Autodesk Inventor part; units mm, degrees
(part 2 of 2)
sketch "Sketch39" plane through (0, 25, 0) normal (0, 1, 0) x (1, 0, 0)
  line L0 (-75.5, 3.9) -> (-75.5, 131.7) projected
  line L1 (0, 3.9) -> (-85.5, 3.9) projected
  line L2 (-75.5, 131.7) -> (-71.5, 131.7)
  line L3 (-71.5, 131.7) -> (-71.5, 3.9)
  line L4 (-71.5, 3.9) -> (-75.5, 3.9)
  line L5 (-75.5, 3.9) -> (-75.5, 131.7)
  line L6 (-10, 3.9) -> (-10, 131.7) projected
  line L7 (-10, 131.7) -> (-14, 131.7)
  line L8 (-14, 131.7) -> (-14, 3.9)
  line L9 (-14, 3.9) -> (-10, 3.9)
  line L10 (-10, 3.9) -> (-10, 131.7)
  line L11 (-59.7793, 8.9543) -> (-63.625, 12.8) projected
  line L12 (-59.7793, 8.9543) -> (-57.7793, 8.9543)
  line L13 (-57.7793, 8.9543) -> (-57.7793, 6.9543)
  line L14 (-57.7793, 6.9543) -> (-59.7793, 6.9543)
  line L15 (-59.7793, 6.9543) -> (-59.7793, 8.9543)
  line L16 (-48.0957, 8.9543) -> (-44.25, 12.8) projected
  line L17 (-48.0957, 8.9543) -> (-50.0957, 8.9543)
  line L18 (-50.0957, 8.9543) -> (-50.0957, 3.9)
  line L19 (-50.0957, 3.9) -> (-48.0957, 3.9)
  line L20 (-48.0957, 3.9) -> (-48.0957, 8.9543)
  line L21 (0, 131.7) -> (-85.5, 131.7) projected
  line L22 (-50.0957, 3.9) -> (-57.7793, 3.9)
  line L23 (-57.7793, 3.9) -> (-57.7793, 131.7)
  line L24 (-57.7793, 131.7) -> (-50.0957, 131.7)
  line L25 (-50.0957, 131.7) -> (-50.0957, 3.9)
  line L26 (-38.4043, 8.9543) -> (-42.25, 12.8) projected
  line L27 (-38.4043, 8.9543) -> (-35.962, 8.9543)
  line L28 (-35.962, 8.9543) -> (-35.962, 3.9)
  line L29 (-35.962, 3.9) -> (-38.4043, 3.9)
  line L30 (-38.4043, 3.9) -> (-38.4043, 8.9543)
  line L31 (-26.7044, 8.9543) -> (-28.7044, 8.9543)
  line L32 (-28.7044, 8.9543) -> (-28.7044, 3.9)
  line L33 (-28.7044, 3.9) -> (-26.7044, 3.9)
  line L34 (-26.7044, 3.9) -> (-26.7044, 8.9543)
  line L35 (-35.962, 3.9) -> (-28.7044, 3.9)
  line L36 (-28.7044, 3.9) -> (-28.7044, 131.7)
  line L37 (-28.7044, 131.7) -> (-35.962, 131.7)
  line L38 (-35.962, 131.7) -> (-35.962, 3.9)
  line L39 (-69.4707, 126.6457) -> (-65.625, 122.8) projected
  line L40 (-69.4707, 126.6457) -> (-71.5, 126.6457)
  line L41 (-71.5, 126.6457) -> (-71.5, 128.6457)
  line L42 (-71.5, 128.6457) -> (-69.4707, 128.6457)
  line L43 (-69.4707, 128.6457) -> (-69.4707, 126.6457)
  line L44 (-85.5, 131.7) -> (-75.5, 131.7) projected
  line L45 (-75.5, 131.7) -> (-10, 131.7)
  line L46 (-10, 131.7) -> (-10, 128.6457)
  line L47 (-10, 128.6457) -> (-75.5, 128.6457)
  line L48 (-75.5, 128.6457) -> (-75.5, 131.7)
  line L49 (-75.5, 3.9) -> (-14, 3.9)
  line L50 (-14, 3.9) -> (-14, 6.9543)
  line L51 (-14, 6.9543) -> (-75.5, 6.9543)
  line L52 (-75.5, 6.9543) -> (-75.5, 3.9)
  point P0 (0, 0)
  point P1 (-28.7044, 128.6457)
  point P2 (-14, 128.6457)
  point P3 (-28.7044, 6.9543)
  point P4 (-50.0957, 128.6457)
  point P5 (-35.962, 128.6457)
  point P6 (-35.962, 6.9543)
  point P7 (-50.0957, 6.9543)
  point P8 (-57.7793, 128.6457)
  point P9 (-71.5, 6.9543)
  dimension "d181" = 4
  dimension "d182" = 4
  dimension "d183" = 2
  dimension "d184" = 2
  dimension "d185" = 2
  dimension "d186" = 2
  dimension "d187" = 2
  constraints: 88 end point, 22 parallel, 14 point on line, 11 horizontal, 11 perpendicular
  measures "d181" distance of L3.end L4.end
  measures "d182" distance of L9.end L8.end
  measures "d183" distance of L13.end L14.end
  measures "d184" distance of L12.end L13.end
  measures "d185" distance of L19.end L18.end
  measures "d186" distance of L33.end L32.end
  measures "d187" distance of L40.end L41.end
extrude "Extrusion36" cut sketch "Sketch39" against normal blind 20 contours L0 L51 L3 L1 | L0 L47 L3 L51 | L3 L51 L14 L23 L1 | L0 L2 L3 L47 | L23 L51 L18 L1 | L3 L21 L23 L47 L42 | L18 L51 L20 L1 | L13 L23 L47 L25 L18 L51 | L20 L51 L30 L1 | L21 L25 L47 L23 | L30 L51 L28 L1 | L21 L38 L47 L25 | L28 L51 L32 L1 | L21 L36 L47 L38 | L47 L36 L32 L51 L28 L38 | L32 L51 L34 L1 | L21 L8 L47 L36 | L34 L51 L8 L1 | L7 L6 L47 L8 | L47 L6 L1 L8
sketch "Sketch41" plane through (0, 25, 0) normal (0, 1, 0) x (1, 0, 0)
  line L0 (-77.7032, 134.0912) -> (-53.8399, 134.0912)
  line L1 (-53.8399, 134.0912) -> (-53.8399, -1.2645)
  line L2 (-53.8399, -1.2645) -> (-77.7032, -1.2645)
  line L3 (-77.7032, -1.2645) -> (-77.7032, 134.0912)
  line L4 (-30.9546, 135.8516) -> (-10.2209, 135.8516)
  line L5 (-10.2209, 135.8516) -> (-10.2209, -6.5457)
  line L6 (-10.2209, -6.5457) -> (-30.9546, -6.5457)
  line L7 (-30.9546, -6.5457) -> (-30.9546, 135.8516)
  point P0 (0, 0)
  constraints: 16 end point, 4 parallel, 2 horizontal, 2 perpendicular
extrude "Extrusion37" cut sketch "Sketch41" against normal blind 20
sketch "Sketch42" plane through (0, 5, 0) normal (0, 1, 0) x (1, 0, 0)
  line L0 (-72.732, 126.4568) -> (-55.877, 126.4568)
  line L1 (-55.877, 126.4568) -> (-55.877, 7.7978)
  line L2 (-55.877, 7.7978) -> (-72.732, 7.7978)
  line L3 (-72.732, 7.7978) -> (-72.732, 126.4568)
  line L4 (-10.2563, 126.4568) -> (-31.3812, 126.4568)
  line L5 (-31.3812, 126.4568) -> (-31.3812, 7.7978)
  line L6 (-31.3812, 7.7978) -> (-10.2563, 7.7978)
  line L7 (-10.2563, 7.7978) -> (-10.2563, 126.4568)
  point P0 (0, 0)
  constraints: 16 end point, 4 parallel, 2 horizontal, 2 perpendicular, 2 point on line
extrude "Extrusion38" add sketch "Sketch42" against normal blind 5
sketch "Sketch43" plane through (0, 5, 0) normal (0, 1, 0) x (1, 0, 0)
  line L0 (0, 131.7) -> (-85.5, 131.7) projected
  line L1 (-85.5, 131.7) -> (-82.446, 131.7)
  line L2 (-82.446, 131.7) -> (-82.446, 128.646)
  line L3 (-82.446, 128.646) -> (-85.5, 128.646)
  line L4 (-85.5, 128.646) -> (-85.5, 131.7)
  line L5 (0, 131.7) -> (-3.054, 131.7)
  line L6 (-3.054, 131.7) -> (-3.054, 128.646)
  line L7 (-3.054, 128.646) -> (0, 128.646)
  line L8 (0, 128.646) -> (0, 131.7)
  line L9 (0, 3.9) -> (-3.054, 3.9)
  line L10 (-3.054, 3.9) -> (-3.054, 6.954)
  line L11 (-3.054, 6.954) -> (0, 6.954)
  line L12 (0, 6.954) -> (0, 3.9)
  line L13 (-85.5, 3.9) -> (-82.446, 3.9)
  line L14 (-82.446, 3.9) -> (-82.446, 6.954)
  line L15 (-82.446, 6.954) -> (-85.5, 6.954)
  line L16 (-85.5, 6.954) -> (-85.5, 3.9)
  line L17 (-82.446, 6.954) -> (-3.054, 6.954)
  line L18 (-3.054, 6.954) -> (-3.054, 128.646)
  line L19 (-3.054, 128.646) -> (-82.446, 128.646)
  line L20 (-82.446, 128.646) -> (-82.446, 6.954)
  line L21 (-82.446, 128.646) -> (-68.312, 128.646)
  line L22 (-68.312, 128.646) -> (-68.312, 6.954)
  line L23 (-68.312, 6.954) -> (-82.446, 6.954)
  line L24 (-82.446, 6.954) -> (-82.446, 128.646)
  line L25 (-3.054, 128.646) -> (-17.188, 128.646)
  line L26 (-17.188, 128.646) -> (-17.188, 6.954)
  line L27 (-17.188, 6.954) -> (-3.054, 6.954)
  line L28 (-3.054, 6.954) -> (-3.054, 128.646)
  point P0 (0, 0)
  dimension "d194" = 3.054
  dimension "d195" = 3.054
  dimension "d196" = 3.054
  dimension "d197" = 3.054
  dimension "d198" = 3.054
  dimension "d199" = 3.054
  dimension "d200" = 3.054
  dimension "d201" = 3.054
  dimension "d202" = 14.134
  dimension "d203" = 14.134
  constraints: 56 end point, 14 parallel, 7 horizontal, 7 perpendicular, 2 point on line
  measures "d194" distance of L2.end L3.end
  measures "d195" distance of L1.end L2.end
  measures "d196" distance of L7.end L6.end
  measures "d197" distance of L6.end L5.end
  measures "d198" distance of L10.end L11.end
  measures "d199" distance of L9.end L10.end
  measures "d200" distance of L15.end L14.end
  measures "d201" distance of L14.end L13.end
  measures "d202" distance of L22.end L23.end
  measures "d203" distance of L27.end L26.end
extrude "Extrusion39" add sketch "Sketch43" along normal blind 20 contours L18 L17 L26 L19 | L19 L22 L17 L20
sketch "Sketch44" plane through (0, 25, 0) normal (0, 1, 0) x (1, 0, 0)
  point P0 (0, 0)
sketch "Sketch45" plane through (0, 25, 0) normal (0, 1, 0) x (1, 0, 0)
  line L0 (-42.25, 22.8) -> (-44.25, 22.8) projected
  line L1 (-2.93, 12.8) -> (-44.25, 12.8)
  line L2 (-44.25, 12.8) -> (-44.25, 22.8)
  line L3 (-44.25, 22.8) -> (-2.93, 22.8)
  line L4 (-2.93, 22.8) -> (-2.93, 12.8)
  line L5 (-42.25, 12.8) -> (-82.5029, 12.8)
  line L6 (-82.5029, 12.8) -> (-82.5029, 22.8)
  line L7 (-82.5029, 22.8) -> (-42.25, 22.8)
  line L8 (-42.25, 22.8) -> (-42.25, 12.8)
  line L9 (-42.25, 32.8) -> (-42.25, 42.8) projected
  line L10 (-42.25, 32.8) -> (-82.5029, 32.8)
  line L11 (-82.5029, 32.8) -> (-82.5029, 42.8)
  line L12 (-82.5029, 42.8) -> (-42.25, 42.8)
  line L13 (-42.25, 42.8) -> (-42.25, 32.8)
  line L14 (-44.25, 42.8) -> (-44.25, 32.8) projected
  line L15 (-3.054, 6.954) -> (-3.054, 128.646) projected
  line L16 (-44.25, 32.8) -> (-3.054, 32.8)
  line L17 (-3.054, 32.8) -> (-3.054, 42.8)
  line L18 (-3.054, 42.8) -> (-44.25, 42.8)
  line L19 (-44.25, 42.8) -> (-44.25, 32.8)
  line L20 (-44.25, 62.8) -> (-44.25, 52.8) projected
  line L21 (-44.25, 52.8) -> (-3.054, 52.8)
  line L22 (-3.054, 52.8) -> (-3.054, 62.8)
  line L23 (-3.054, 62.8) -> (-44.25, 62.8)
  line L24 (-44.25, 62.8) -> (-44.25, 52.8)
  line L25 (-44.25, 52.8) -> (-42.25, 52.8) projected
  line L26 (-42.25, 52.8) -> (-82.5029, 52.8)
  line L27 (-82.5029, 52.8) -> (-82.5029, 62.8)
  line L28 (-82.5029, 62.8) -> (-42.25, 62.8)
  line L29 (-42.25, 62.8) -> (-42.25, 52.8)
  line L30 (-44.25, 72.8) -> (-42.25, 72.8) projected
  line L31 (-44.25, 72.8) -> (-3.054, 72.8)
  line L32 (-3.054, 72.8) -> (-3.054, 82.8104)
  line L33 (-3.054, 82.8104) -> (-44.25, 82.8104)
  line L34 (-44.25, 82.8104) -> (-44.25, 72.8)
  line L35 (-42.25, 72.8) -> (-42.25, 82.8) projected
  line L36 (-42.25, 72.8) -> (-82.5029, 72.8)
  line L37 (-82.5029, 72.8) -> (-82.5029, 82.8104)
  line L38 (-82.5029, 82.8104) -> (-42.25, 82.8104)
  line L39 (-42.25, 82.8104) -> (-42.25, 72.8)
  line L40 (-44.25, 102.8) -> (-44.25, 92.8) projected
  line L41 (-44.25, 92.8) -> (-3.054, 92.8)
  line L42 (-3.054, 92.8) -> (-3.054, 102.8)
  line L43 (-3.054, 102.8) -> (-44.25, 102.8)
  line L44 (-44.25, 102.8) -> (-44.25, 92.8)
  line L45 (-42.25, 92.8) -> (-42.25, 102.8) projected
  line L46 (-82.446, 6.954) -> (-82.446, 128.646) projected
  line L47 (-42.25, 92.8) -> (-82.446, 92.8)
  line L48 (-82.446, 92.8) -> (-82.446, 102.8)
  line L49 (-82.446, 102.8) -> (-42.25, 102.8)
  line L50 (-42.25, 102.8) -> (-42.25, 92.8)
  line L51 (-42.25, 112.8) -> (-82.446, 112.8)
  line L52 (-82.446, 112.8) -> (-82.446, 122.8)
  line L53 (-82.446, 122.8) -> (-42.25, 122.8)
  line L54 (-42.25, 122.8) -> (-42.25, 112.8)
  line L55 (-44.25, 112.8) -> (-3.054, 112.8)
  line L56 (-3.054, 112.8) -> (-3.054, 122.8)
  line L57 (-3.054, 122.8) -> (-44.25, 122.8)
  line L58 (-44.25, 122.8) -> (-44.25, 112.8)
  line L59 (-17.188, 128.646) -> (-17.188, 6.954) projected
  line L60 (-3.054, 128.646) -> (-17.188, 128.646) projected
  line L61 (-17.188, 6.954) -> (-11.324, 6.954)
  line L62 (-11.324, 6.954) -> (-11.324, 128.646)
  line L63 (-11.324, 128.646) -> (-17.188, 128.646)
  line L64 (-17.188, 128.646) -> (-17.188, 6.954)
  line L65 (-82.446, 6.954) -> (-68.312, 6.954) projected
  line L66 (-68.312, 128.646) -> (-82.446, 128.646) projected
  line L67 (-68.312, 6.954) -> (-74.176, 6.954)
  line L68 (-74.176, 6.954) -> (-74.176, 128.646)
  line L69 (-74.176, 128.646) -> (-68.312, 128.646)
  line L70 (-68.312, 128.646) -> (-68.312, 6.954)
  line L71 (-82.446, 128.646) -> (-76.582, 128.646)
  line L72 (-76.582, 128.646) -> (-76.582, 6.954)
  line L73 (-76.582, 6.954) -> (-82.446, 6.954)
  line L74 (-82.446, 6.954) -> (-82.446, 128.646)
  line L75 (-17.188, 6.954) -> (-3.054, 6.954) projected
  line L76 (-3.054, 6.954) -> (-8.918, 6.954)
  line L77 (-8.918, 6.954) -> (-8.918, 128.646)
  line L78 (-8.918, 128.646) -> (-3.054, 128.646)
  line L79 (-3.054, 128.646) -> (-3.054, 6.954)
  point P0 (0, 0)
  point P1 (-76.582, 22.8)
  point P2 (-76.582, 12.8)
  point P3 (-74.176, 12.8)
  point P4 (-74.176, 22.8)
  point P5 (-76.582, 42.8)
  point P6 (-76.582, 32.8)
  point P7 (-74.176, 32.8)
  point P8 (-74.176, 42.8)
  point P9 (-76.582, 62.8)
  point P10 (-76.582, 52.8)
  point P11 (-74.176, 52.8)
  point P12 (-74.176, 62.8)
  point P13 (-76.582, 82.8104)
  point P14 (-76.582, 72.8)
  point P15 (-74.176, 72.8)
  point P16 (-74.176, 82.8104)
  point P17 (-76.582, 102.8)
  point P18 (-76.582, 92.8)
  point P19 (-74.176, 92.8)
  point P20 (-74.176, 102.8)
  point P21 (-76.582, 122.8)
  point P22 (-76.582, 112.8)
  point P23 (-74.176, 112.8)
  point P24 (-74.176, 122.8)
  point P25 (-8.918, 112.8)
  point P26 (-8.918, 122.8)
  point P27 (-11.324, 122.8)
  point P28 (-11.324, 112.8)
  point P29 (-8.918, 92.8)
  point P30 (-8.918, 102.8)
  point P31 (-11.324, 102.8)
  point P32 (-11.324, 92.8)
  point P33 (-8.918, 72.8)
  point P34 (-8.918, 82.8104)
  point P35 (-11.324, 82.8104)
  point P36 (-11.324, 72.8)
  point P37 (-8.918, 52.8)
  point P38 (-8.918, 62.8)
  point P39 (-11.324, 62.8)
  point P40 (-11.324, 52.8)
  point P41 (-8.918, 32.8)
  point P42 (-8.918, 42.8)
  point P43 (-11.324, 42.8)
  point P44 (-11.324, 32.8)
  point P45 (-8.918, 12.8)
  point P46 (-8.918, 22.8)
  point P47 (-11.324, 22.8)
  point P48 (-11.324, 12.8)
  dimension "d206" = 5.864
  dimension "d207" = 5.864
  dimension "d208" = 5.864
  dimension "d209" = 5.864
  constraints: 128 end point, 32 parallel, 21 point on line, 16 horizontal, 16 perpendicular
  measures "d206" distance of L63.end L62.end
  measures "d207" distance of L68.end L69.end
  measures "d208" distance of L72.end L73.end
  measures "d209" distance of L77.end L78.end
extrude "Extrusion40" cut sketch "Sketch45" against normal blind 100 contours L3 L77 L1 L62 | L68 L5 L72 L7 | L62 L18 L77 L16 | L10 L72 L12 L68 | L62 L23 L77 L21 | L26 L72 L28 L68 | L62 L33 L77 L31 | L36 L72 L38 L68 | L62 L43 L77 L41 | L47 L72 L49 L68 | L62 L57 L77 L55 | L51 L72 L53 L68
chamfer "Chamfer6" distance 5 distance2 15 1 edges at (-8.918, 25, -17.8) measured on face at (-8.418, 25, -17.8)
chamfer "Chamfer7" distance 5 distance2 15 1 edges at (-8.918, 25, -37.8) measured on face at (-8.418, 25, -37.8)
chamfer "Chamfer8" distance 5 distance2 15 1 edges at (-8.918, 25, -57.8) measured on face at (-8.418, 25, -57.8)
chamfer "Chamfer9" distance 5 distance2 15 1 edges at (-8.918, 25, -77.8052) measured on face at (-8.418, 25, -77.8052)
chamfer "Chamfer10" distance 5 distance2 15 1 edges at (-8.918, 25, -97.8) measured on face at (-8.418, 25, -97.8)
chamfer "Chamfer11" distance 5 distance2 15 1 edges at (-8.918, 25, -117.8) measured on face at (-8.418, 25, -117.8)
chamfer "Chamfer12" distance 5 distance2 15 1 edges at (-11.324, 25, -117.8) measured on face at (-11.824, 25, -117.8)
chamfer "Chamfer13" distance 5 distance2 15 1 edges at (-11.324, 25, -97.8) measured on face at (-11.824, 25, -97.8)
chamfer "Chamfer14" distance 5 distance2 15 1 edges at (-11.324, 25, -77.8052) measured on face at (-11.824, 25, -77.8052)
chamfer "Chamfer15" distance 5 distance2 15 1 edges at (-11.324, 25, -57.8) measured on face at (-11.824, 25, -57.8)
chamfer "Chamfer16" distance 5 distance2 15 1 edges at (-11.324, 25, -37.8) measured on face at (-11.824, 25, -37.8)
chamfer "Chamfer17" distance 5 distance2 15 1 edges at (-11.324, 25, -17.8) measured on face at (-11.824, 25, -17.8)
chamfer "Chamfer18" distance 5 distance2 15 1 edges at (-74.176, 25, -17.8) measured on face at (-73.676, 25, -17.8)
chamfer "Chamfer19" distance 5 distance2 15 1 edges at (-76.582, 25, -17.8) measured on face at (-77.082, 25, -17.8)
chamfer "Chamfer20" distance 5 distance2 15 1 edges at (-74.176, 25, -37.8) measured on face at (-73.676, 25, -37.8)
chamfer "Chamfer21" distance 5 distance2 15 1 edges at (-76.582, 25, -37.8) measured on face at (-77.082, 25, -37.8)
chamfer "Chamfer22" distance 5 distance2 15 1 edges at (-76.582, 25, -57.8) measured on face at (-77.082, 25, -57.8)
chamfer "Chamfer23" distance 5 distance2 15 1 edges at (-74.176, 25, -57.8) measured on face at (-73.676, 25, -57.8)
chamfer "Chamfer24" distance 5 distance2 15 1 edges at (-74.176, 25, -77.8052) measured on face at (-73.676, 25, -77.8052)
chamfer "Chamfer25" distance 5 distance2 15 1 edges at (-76.582, 25, -77.8052) measured on face at (-77.082, 25, -77.8052)
chamfer "Chamfer26" distance 5 distance2 15 1 edges at (-74.176, 25, -97.8) measured on face at (-73.676, 25, -97.8)
chamfer "Chamfer27" distance 5 distance2 15 1 edges at (-76.582, 25, -97.8) measured on face at (-77.082, 25, -97.8)
chamfer "Chamfer28" distance 5 distance2 15 1 edges at (-74.176, 25, -117.8) measured on face at (-73.676, 25, -117.8)
chamfer "Chamfer29" distance 5 distance2 15 1 edges at (-76.582, 25, -117.8) measured on face at (-77.082, 25, -117.8)
chamfer "Chamfer30" distance 1 distance2 15 3 edges at (-13.824, 25, -12.8) (-10.121, 25, -12.8) (-6.418, 25, -12.8) measured on face at (-13.824, 25, -12.3) measured on face at (-10.121, 25, -12.3) measured on face at (-6.418, 25, -12.3)
chamfer "Chamfer31" distance 1 distance2 15 3 edges at (-6.418, 25, -22.8) (-10.121, 25, -22.8) (-13.824, 25, -22.8) measured on face at (-13.824, 25, -23.3) measured on face at (-10.121, 25, -23.3) measured on face at (-6.418, 25, -23.3)
chamfer "Chamfer32" distance 1 distance2 15 3 edges at (-13.824, 25, -32.8) (-10.121, 25, -32.8) (-6.418, 25, -32.8) measured on face at (-10.121, 25, -32.3) measured on face at (-6.418, 25, -32.3) measured on face at (-13.824, 25, -32.3)
chamfer "Chamfer33" distance 1 distance2 15 3 edges at (-6.418, 25, -42.8) (-10.121, 25, -42.8) (-13.824, 25, -42.8) measured on face at (-10.121, 25, -43.3) measured on face at (-6.418, 25, -43.3) measured on face at (-13.824, 25, -43.3)
chamfer "Chamfer34" distance 1 distance2 15 3 edges at (-13.824, 25, -62.8) (-10.121, 25, -62.8) (-6.418, 25, -62.8) measured on face at (-6.418, 25, -63.3) measured on face at (-13.824, 25, -63.3) measured on face at (-10.121, 25, -63.3)
chamfer "Chamfer35" distance 1 distance2 15 3 edges at (-6.418, 25, -52.8) (-10.121, 25, -52.8) (-13.824, 25, -52.8) measured on face at (-6.418, 25, -52.3) measured on face at (-13.824, 25, -52.3) measured on face at (-10.121, 25, -52.3)
chamfer "Chamfer36" distance 1 distance2 15 3 edges at (-13.824, 25, -72.8) (-10.121, 25, -72.8) (-6.418, 25, -72.8) measured on face at (-6.418, 25, -72.3) measured on face at (-13.824, 25, -72.3) measured on face at (-10.121, 25, -72.3)
chamfer "Chamfer37" distance 1 distance2 15 3 edges at (-6.418, 25, -82.8104) (-10.121, 25, -82.8104) (-13.824, 25, -82.8104) measured on face at (-13.824, 25, -83.3104) measured on face at (-10.121, 25, -83.3104) measured on face at (-6.418, 25, -83.3104)
chamfer "Chamfer38" distance 1 distance2 15 3 edges at (-13.824, 25, -92.8) (-10.121, 25, -92.8) (-6.418, 25, -92.8) measured on face at (-13.824, 25, -92.3) measured on face at (-10.121, 25, -92.3) measured on face at (-6.418, 25, -92.3)
chamfer "Chamfer39" distance 1 distance2 15 3 edges at (-6.418, 25, -102.8) (-10.121, 25, -102.8) (-13.824, 25, -102.8) measured on face at (-13.824, 25, -103.3) measured on face at (-10.121, 25, -103.3) measured on face at (-6.418, 25, -103.3)
chamfer "Chamfer40" distance 1 distance2 15 3 edges at (-13.824, 25, -112.8) (-10.121, 25, -112.8) (-6.418, 25, -112.8) measured on face at (-6.418, 25, -112.3) measured on face at (-13.824, 25, -112.3) measured on face at (-10.121, 25, -112.3)
chamfer "Chamfer41" distance 1 distance2 15 3 edges at (-6.418, 25, -122.8) (-10.121, 25, -122.8) (-13.824, 25, -122.8) measured on face at (-6.418, 25, -123.3) measured on face at (-13.824, 25, -123.3) measured on face at (-10.121, 25, -123.3)
chamfer "Chamfer42" distance 1 distance2 15 3 edges at (-79.082, 25, -12.8) (-75.379, 25, -12.8) (-71.676, 25, -12.8) measured on face at (-75.379, 25, -12.3) measured on face at (-71.676, 25, -12.3) measured on face at (-79.082, 25, -12.3)
chamfer "Chamfer43" distance 1 distance2 15 3 edges at (-71.676, 25, -22.8) (-75.379, 25, -22.8) (-79.082, 25, -22.8) measured on face at (-75.379, 25, -23.3) measured on face at (-71.676, 25, -23.3) measured on face at (-79.082, 25, -23.3)
chamfer "Chamfer44" distance 1 distance2 15 3 edges at (-79.082, 25, -42.8) (-75.379, 25, -42.8) (-71.676, 25, -42.8) measured on face at (-71.676, 25, -43.3) measured on face at (-75.379, 25, -43.3) measured on face at (-79.082, 25, -43.3)
chamfer "Chamfer45" distance 1 distance2 15 3 edges at (-71.676, 25, -32.8) (-75.379, 25, -32.8) (-79.082, 25, -32.8) measured on face at (-75.379, 25, -32.3) measured on face at (-71.676, 25, -32.3) measured on face at (-79.082, 25, -32.3)
chamfer "Chamfer46" distance 1 distance2 15 3 edges at (-71.676, 25, -52.8) (-75.379, 25, -52.8) (-79.082, 25, -52.8) measured on face at (-71.676, 25, -52.3) measured on face at (-75.379, 25, -52.3) measured on face at (-79.082, 25, -52.3)
chamfer "Chamfer47" distance 1 distance2 15 3 edges at (-79.082, 25, -62.8) (-75.379, 25, -62.8) (-71.676, 25, -62.8) measured on face at (-71.676, 25, -63.3) measured on face at (-75.379, 25, -63.3) measured on face at (-79.082, 25, -63.3)
chamfer "Chamfer48" distance 1 distance2 15 3 edges at (-79.082, 25, -72.8) (-75.379, 25, -72.8) (-71.676, 25, -72.8) measured on face at (-71.676, 25, -72.3) measured on face at (-75.379, 25, -72.3) measured on face at (-79.082, 25, -72.3)
chamfer "Chamfer49" distance 1 distance2 15 3 edges at (-71.676, 25, -82.8104) (-75.379, 25, -82.8104) (-79.082, 25, -82.8104) measured on face at (-71.676, 25, -83.3104) measured on face at (-79.082, 25, -83.3104) measured on face at (-75.379, 25, -83.3104)
chamfer "Chamfer50" distance 1 distance2 15 3 edges at (-79.082, 25, -92.8) (-75.379, 25, -92.8) (-71.676, 25, -92.8) measured on face at (-71.676, 25, -92.3) measured on face at (-75.379, 25, -92.3) measured on face at (-79.082, 25, -92.3)
chamfer "Chamfer51" distance 1 distance2 15 3 edges at (-71.676, 25, -102.8) (-75.379, 25, -102.8) (-79.082, 25, -102.8) measured on face at (-75.379, 25, -103.3) measured on face at (-71.676, 25, -103.3) measured on face at (-79.082, 25, -103.3)
chamfer "Chamfer52" distance 1 distance2 15 3 edges at (-79.082, 25, -112.8) (-75.379, 25, -112.8) (-71.676, 25, -112.8) measured on face at (-75.379, 25, -112.3) measured on face at (-79.082, 25, -112.3) measured on face at (-71.676, 25, -112.3)
chamfer "Chamfer53" distance 1 distance2 15 3 edges at (-71.676, 25, -122.8) (-75.379, 25, -122.8) (-79.082, 25, -122.8) measured on face at (-75.379, 25, -123.3) measured on face at (-79.082, 25, -123.3) measured on face at (-71.676, 25, -123.3)
sketch "Sketch46" plane through (0, 25, 0) normal (0, 1, 0) x (1, 0, 0)
  line L0 (-42.25, 12.8) -> (-42.25, 22.8) projected
  line L1 (-42.25, 22.8) -> (-44.25, 22.8) projected
  line L2 (-42.25, 12.8) -> (-44.25, 12.8)
  line L3 (-44.25, 12.8) -> (-44.25, 22.8)
  line L4 (-44.25, 22.8) -> (-42.25, 22.8)
  line L5 (-42.25, 22.8) -> (-42.25, 12.8)
  line L6 (-44.25, 32.8) -> (-42.25, 32.8) projected
  line L7 (-42.25, 42.8) -> (-44.25, 42.8) projected
  line L8 (-42.25, 32.8) -> (-44.25, 32.8)
  line L9 (-44.25, 32.8) -> (-44.25, 42.8)
  line L10 (-44.25, 42.8) -> (-42.25, 42.8)
  line L11 (-42.25, 42.8) -> (-42.25, 32.8)
  line L12 (-42.25, 52.8) -> (-42.25, 62.8) projected
  line L13 (-42.25, 52.8) -> (-44.25, 52.8)
  line L14 (-44.25, 52.8) -> (-44.25, 62.8)
  line L15 (-44.25, 62.8) -> (-42.25, 62.8)
  line L16 (-42.25, 62.8) -> (-42.25, 52.8)
  line L17 (-42.25, 72.8) -> (-42.25, 82.8) projected
  line L18 (-42.25, 72.8) -> (-44.25, 72.8)
  line L19 (-44.25, 72.8) -> (-44.25, 82.8)
  line L20 (-44.25, 82.8) -> (-42.25, 82.8)
  line L21 (-42.25, 82.8) -> (-42.25, 72.8)
  line L22 (-42.25, 92.8098) -> (-44.25, 92.8098)
  line L23 (-44.25, 92.8098) -> (-44.25, 102.7913)
  line L24 (-44.25, 102.7913) -> (-42.25, 102.7913)
  line L25 (-42.25, 102.7913) -> (-42.25, 92.8098)
  line L26 (-42.25, 112.8) -> (-42.25, 122.8) projected
  line L27 (-42.25, 112.8) -> (-44.25, 112.8)
  line L28 (-44.25, 112.8) -> (-44.25, 122.8)
  line L29 (-44.25, 122.8) -> (-42.25, 122.8)
  line L30 (-42.25, 122.8) -> (-42.25, 112.8)
  point P0 (0, 0)
  constraints: 48 end point, 12 parallel, 6 horizontal, 6 perpendicular, 5 point on line
sketch "Sketch47" plane through (0, 25, 0) normal (0, 1, 0) x (1, 0, 0)
  line L0 (-35.962, 6.9543) -> (-35.962, 128.6457) projected
  line L1 (-50.0957, 128.6457) -> (-50.0957, 6.9543) projected
  line L2 (-35.962, 6.9543) -> (-50.0957, 6.9543)
  line L3 (-50.0957, 6.9543) -> (-50.0957, 128.6457)
  line L4 (-50.0957, 128.6457) -> (-35.962, 128.6457)
  line L5 (-35.962, 128.6457) -> (-35.962, 6.9543)
  point P0 (0, 0)
  constraints: 8 end point, 2 parallel, 1 horizontal, 1 perpendicular
extrude "Extrusion41" add sketch "Sketch47" against normal blind 25
extrude "Extrusion42" cut sketch "Sketch46" against normal blind 25
chamfer "Chamfer54" distance 5 distance2 15 1 edges at (-44.25, 25, -17.8) measured on face at (-44.75, 25, -17.8)
chamfer "Chamfer55" distance 5 distance2 15 1 edges at (-42.25, 25, -17.8) measured on face at (-41.75, 25, -17.8)
chamfer "Chamfer56" distance 5 distance2 15 1 edges at (-42.25, 25, -37.8) measured on face at (-41.75, 25, -37.8)
chamfer "Chamfer57" distance 5 distance2 15 1 edges at (-44.25, 25, -37.8) measured on face at (-44.75, 25, -37.8)
chamfer "Chamfer58" distance 5 distance2 15 1 edges at (-42.25, 25, -57.8) measured on face at (-41.75, 25, -57.8)
chamfer "Chamfer59" distance 5 distance2 15 1 edges at (-44.25, 25, -57.8) measured on face at (-44.75, 25, -57.8)
chamfer "Chamfer60" distance 5 distance2 15 1 edges at (-42.25, 25, -77.8) measured on face at (-41.75, 25, -77.8)
chamfer "Chamfer61" distance 5 distance2 15 1 edges at (-44.25, 25, -77.8) measured on face at (-44.75, 25, -77.8)
chamfer "Chamfer62" distance 5 distance2 15 1 edges at (-42.25, 25, -97.8005)
chamfer "Chamfer63" distance 5 distance2 15 1 edges at (-44.25, 25, -97.8005)
chamfer "Chamfer64" distance 5 distance2 15 1 edges at (-42.25, 25, -117.8) measured on face at (-41.75, 25, -117.8)
chamfer "Chamfer65" distance 5 distance2 15 1 edges at (-44.25, 25, -117.8) measured on face at (-44.75, 25, -117.8)
chamfer "Chamfer66" distance 1 distance2 15 3 edges at (-39.75, 25, -12.8) (-43.25, 25, -12.8) (-46.75, 25, -12.8) measured on face at (-43.25, 25, -12.3) measured on face at (-46.75, 25, -12.3) measured on face at (-39.75, 25, -12.3)
chamfer "Chamfer67" distance 1 distance2 15 3 edges at (-46.75, 25, -22.8) (-43.25, 25, -22.8) (-39.75, 25, -22.8) measured on face at (-39.75, 25, -23.3) measured on face at (-46.75, 25, -23.3) measured on face at (-43.25, 25, -23.3)
chamfer "Chamfer68" distance 1 distance2 15 3 edges at (-46.75, 25, -32.8) (-43.25, 25, -32.8) (-39.75, 25, -32.8) measured on face at (-46.75, 25, -32.3) measured on face at (-43.25, 25, -32.3) measured on face at (-39.75, 25, -32.3)
chamfer "Chamfer69" distance 1 distance2 15 3 edges at (-39.75, 25, -42.8) (-43.25, 25, -42.8) (-46.75, 25, -42.8) measured on face at (-46.75, 25, -43.3) measured on face at (-43.25, 25, -43.3) measured on face at (-39.75, 25, -43.3)
chamfer "Chamfer70" distance 1 distance2 15 3 edges at (-46.75, 25, -52.8) (-43.25, 25, -52.8) (-39.75, 25, -52.8) measured on face at (-43.25, 25, -52.3) measured on face at (-39.75, 25, -52.3) measured on face at (-46.75, 25, -52.3)
chamfer "Chamfer71" distance 1 distance2 15 3 edges at (-46.75, 25, -72.8) (-43.25, 25, -72.8) (-39.75, 25, -72.8) measured on face at (-46.75, 25, -72.3) measured on face at (-43.25, 25, -72.3) measured on face at (-39.75, 25, -72.3)
chamfer "Chamfer72" distance 1 distance2 15 3 edges at (-39.75, 25, -62.8) (-43.25, 25, -62.8) (-46.75, 25, -62.8) measured on face at (-39.75, 25, -63.3) measured on face at (-43.25, 25, -63.3) measured on face at (-46.75, 25, -63.3)
chamfer "Chamfer73" distance 1 distance2 15 3 edges at (-39.75, 25, -82.8) (-43.25, 25, -82.8) (-46.75, 25, -82.8) measured on face at (-46.75, 25, -83.3) measured on face at (-43.25, 25, -83.3) measured on face at (-39.75, 25, -83.3)
chamfer "Chamfer74" distance 1 distance2 15 3 edges at (-39.75, 25, -92.8098) (-46.75, 25, -92.8098) (-43.25, 25, -92.8098) measured on face at (-46.75, 25, -92.3098) measured on face at (-43.5833, 25, -92.8066) measured on face at (-39.75, 25, -92.3098)
chamfer "Chamfer75" distance 1 distance2 15 3 edges at (-46.75, 25, -102.7913) (-39.75, 25, -102.7913) (-43.25, 25, -102.7913) measured on face at (-39.75, 25, -103.2913) measured on face at (-43.5833, 25, -102.7971) measured on face at (-46.75, 25, -103.2913)
chamfer "Chamfer76" distance 1 distance2 15 3 edges at (-46.75, 25, -112.8) (-43.25, 25, -112.8) (-39.75, 25, -112.8) measured on face at (-46.75, 25, -112.3) measured on face at (-43.25, 25, -112.3) measured on face at (-39.75, 25, -112.3)
chamfer "Chamfer77" distance 1 distance2 15 3 edges at (-39.75, 25, -122.8) (-43.25, 25, -122.8) (-46.75, 25, -122.8) measured on face at (-46.75, 25, -123.3) measured on face at (-43.25, 25, -123.3) measured on face at (-39.75, 25, -123.3)
chamfer "Chamfer78" distance 5 distance2 2 3 edges at (-79.082, 25, -11.8) (-75.379, 25, -11.8) (-71.676, 25, -11.8) measured on face at (-71.676, 24.5011, -11.8333) measured on face at (-75.379, 24.5011, -11.8333) measured on face at (-79.082, 24.5011, -11.8333)
chamfer "Chamfer79" distance 5 distance2 2 3 edges at (-71.676, 25, -23.8) (-75.379, 25, -23.8) (-79.082, 25, -23.8) measured on face at (-79.082, 24.5011, -23.7667) measured on face at (-75.379, 24.5011, -23.7667) measured on face at (-71.676, 24.5011, -23.7667)
chamfer "Chamfer80" distance 5 distance2 2 3 edges at (-79.082, 25, -31.8) (-75.379, 25, -31.8) (-71.676, 25, -31.8) measured on face at (-71.676, 24.5011, -31.8333) measured on face at (-75.379, 24.5011, -31.8333) measured on face at (-79.082, 24.5011, -31.8333)
chamfer "Chamfer81" distance 5 distance2 2 3 edges at (-79.082, 25, -43.8) (-75.379, 25, -43.8) (-71.676, 25, -43.8) measured on face at (-71.676, 24.5011, -43.7667) measured on face at (-75.379, 24.5011, -43.7667) measured on face at (-79.082, 24.5011, -43.7667)
chamfer "Chamfer82" distance 5 distance2 2 3 edges at (-71.676, 25, -51.8) (-75.379, 25, -51.8) (-79.082, 25, -51.8) measured on face at (-71.676, 24.5011, -51.8333) measured on face at (-79.082, 24.5011, -51.8333) measured on face at (-75.379, 24.5011, -51.8333)
chamfer "Chamfer83" distance 5 distance2 2 3 edges at (-79.082, 25, -63.8) (-75.379, 25, -63.8) (-71.676, 25, -63.8) measured on face at (-71.676, 24.5011, -63.7667) measured on face at (-75.379, 24.5011, -63.7667) measured on face at (-79.082, 24.5011, -63.7667)
chamfer "Chamfer84" distance 5 distance2 2 3 edges at (-79.082, 25, -71.8) (-75.379, 25, -71.8) (-71.676, 25, -71.8) measured on face at (-75.379, 24.5011, -71.8333) measured on face at (-79.082, 24.5011, -71.8333) measured on face at (-71.676, 24.5011, -71.8333)
chamfer "Chamfer85" distance 5 distance2 2 3 edges at (-71.676, 25, -83.8104) (-75.379, 25, -83.8104) (-79.082, 25, -83.8104) measured on face at (-71.676, 24.5011, -83.7771) measured on face at (-75.379, 24.5011, -83.7771) measured on face at (-79.082, 24.5011, -83.7771)
chamfer "Chamfer86" distance 5 distance2 2 3 edges at (-79.082, 25, -91.8) (-75.379, 25, -91.8) (-71.676, 25, -91.8) measured on face at (-71.676, 24.5011, -91.8333) measured on face at (-75.379, 24.5011, -91.8333) measured on face at (-79.082, 24.5011, -91.8333)
chamfer "Chamfer87" distance 5 distance2 2 3 edges at (-71.676, 25, -103.8) (-75.379, 25, -103.8) (-79.082, 25, -103.8) measured on face at (-71.676, 24.5011, -103.7667) measured on face at (-75.379, 24.5011, -103.7667) measured on face at (-79.082, 24.5011, -103.7667)
chamfer "Chamfer88" distance 5 distance2 2 3 edges at (-79.082, 25, -111.8) (-75.379, 25, -111.8) (-71.676, 25, -111.8) measured on face at (-75.379, 24.5011, -111.8333) measured on face at (-71.676, 24.5011, -111.8333) measured on face at (-79.082, 24.5011, -111.8333)
chamfer "Chamfer89" distance 5 distance2 2 3 edges at (-71.676, 25, -123.8) (-75.379, 25, -123.8) (-79.082, 25, -123.8) measured on face at (-71.676, 24.5011, -123.7667) measured on face at (-75.379, 24.5011, -123.7667) measured on face at (-79.082, 24.5011, -123.7667)
chamfer "Chamfer90" distance 5 distance2 2 3 edges at (-39.75, 25, -11.8) (-43.25, 25, -11.8) (-46.75, 25, -11.8) measured on face at (-46.75, 24.5011, -11.8333) measured on face at (-43.25, 24.5011, -11.8333) measured on face at (-39.75, 24.5011, -11.8333)
chamfer "Chamfer91" distance 5 distance2 2 3 edges at (-46.75, 25, -23.8) (-43.25, 25, -23.8) (-39.75, 25, -23.8) measured on face at (-46.75, 24.5011, -23.7667) measured on face at (-43.25, 24.5011, -23.7667) measured on face at (-39.75, 24.5011, -23.7667)
chamfer "Chamfer92" distance 5 distance2 2 3 edges at (-46.75, 25, -31.8) (-43.25, 25, -31.8) (-39.75, 25, -31.8) measured on face at (-43.25, 24.5011, -31.8333) measured on face at (-39.75, 24.5011, -31.8333) measured on face at (-46.75, 24.5011, -31.8333)
chamfer "Chamfer93" distance 5 distance2 2 3 edges at (-39.75, 25, -43.8) (-43.25, 25, -43.8) (-46.75, 25, -43.8) measured on face at (-46.75, 24.5011, -43.7667) measured on face at (-43.25, 24.5011, -43.7667) measured on face at (-39.75, 24.5011, -43.7667)
chamfer "Chamfer94" distance 5 distance2 2 3 edges at (-46.75, 25, -51.8) (-43.25, 25, -51.8) (-39.75, 25, -51.8) measured on face at (-46.75, 24.5011, -51.8333) measured on face at (-43.25, 24.5011, -51.8333) measured on face at (-39.75, 24.5011, -51.8333)
chamfer "Chamfer95" distance 5 distance2 2 3 edges at (-39.75, 25, -63.8) (-43.25, 25, -63.8) (-46.75, 25, -63.8) measured on face at (-43.25, 24.5011, -63.7667) measured on face at (-39.75, 24.5011, -63.7667) measured on face at (-46.75, 24.5011, -63.7667)
chamfer "Chamfer96" distance 5 distance2 2 3 edges at (-46.75, 25, -71.8) (-43.25, 25, -71.8) (-39.75, 25, -71.8) measured on face at (-46.75, 24.5011, -71.8333) measured on face at (-43.25, 24.5011, -71.8333) measured on face at (-39.75, 24.5011, -71.8333)
chamfer "Chamfer97" distance 5 distance2 2 3 edges at (-39.75, 25, -83.8) (-43.25, 25, -83.8) (-46.75, 25, -83.8) measured on face at (-46.75, 24.5011, -83.7667) measured on face at (-43.25, 24.5011, -83.7667) measured on face at (-39.75, 24.5011, -83.7667)
chamfer "Chamfer98" distance 5 distance2 2 3 edges at (-39.75, 25, -91.8099) (-43.25, 25, -91.8099) (-46.75, 25, -91.8099) measured on face at (-43.25, 24.5011, -91.8432) measured on face at (-39.75, 24.5011, -91.8432) measured on face at (-46.75, 24.5011, -91.8432)
chamfer "Chamfer99" distance 5 distance2 2 3 edges at (-46.75, 25, -103.7912) (-43.25, 25, -103.7912) (-39.75, 25, -103.7912) measured on face at (-46.75, 24.5011, -103.7579) measured on face at (-43.25, 24.5011, -103.7579) measured on face at (-39.75, 24.5011, -103.7579)
chamfer "Chamfer100" distance 5 distance2 2 3 edges at (-46.75, 25, -111.8) (-43.25, 25, -111.8) (-39.75, 25, -111.8) measured on face at (-46.75, 24.5011, -111.8333) measured on face at (-43.25, 24.5011, -111.8333) measured on face at (-39.75, 24.5011, -111.8333)
chamfer "Chamfer101" distance 5 distance2 2 3 edges at (-39.75, 25, -123.8) (-43.25, 25, -123.8) (-46.75, 25, -123.8) measured on face at (-46.75, 24.5011, -123.7667) measured on face at (-39.75, 24.5011, -123.7667) measured on face at (-43.25, 24.5011, -123.7667)
chamfer "Chamfer102" distance 5 distance2 2 3 edges at (-13.824, 25, -11.8) (-10.121, 25, -11.8) (-6.418, 25, -11.8) measured on face at (-13.824, 24.5011, -11.8333) measured on face at (-10.121, 24.5011, -11.8333) measured on face at (-6.418, 24.5011, -11.8333)
chamfer "Chamfer103" distance 5 distance2 2 3 edges at (-6.418, 25, -23.8) (-10.121, 25, -23.8) (-13.824, 25, -23.8) measured on face at (-6.418, 24.5011, -23.7667) measured on face at (-13.824, 24.5011, -23.7667) measured on face at (-10.121, 24.5011, -23.7667)
chamfer "Chamfer104" distance 5 distance2 2 3 edges at (-13.824, 25, -31.8) (-10.121, 25, -31.8) (-6.418, 25, -31.8) measured on face at (-10.121, 24.5011, -31.8333) measured on face at (-13.824, 24.5011, -31.8333) measured on face at (-6.418, 24.5011, -31.8333)
chamfer "Chamfer105" distance 5 distance2 2 3 edges at (-6.418, 25, -43.8) (-10.121, 25, -43.8) (-13.824, 25, -43.8) measured on face at (-13.824, 24.5011, -43.7667) measured on face at (-10.121, 24.5011, -43.7667) measured on face at (-6.418, 24.5011, -43.7667)
chamfer "Chamfer106" distance 5 distance2 2 3 edges at (-13.824, 25, -51.8) (-10.121, 25, -51.8) (-6.418, 25, -51.8) measured on face at (-6.418, 24.5011, -51.8333) measured on face at (-13.824, 24.5011, -51.8333) measured on face at (-10.121, 24.5011, -51.8333)
chamfer "Chamfer107" distance 5 distance2 2 3 edges at (-13.824, 25, -63.8) (-10.121, 25, -63.8) (-6.418, 25, -63.8) measured on face at (-6.418, 24.5011, -63.7667) measured on face at (-13.824, 24.5011, -63.7667) measured on face at (-10.121, 24.5011, -63.7667)
chamfer "Chamfer108" distance 5 distance2 2 3 edges at (-13.824, 25, -71.8) (-10.121, 25, -71.8) (-6.418, 25, -71.8) measured on face at (-10.121, 24.5011, -71.8333) measured on face at (-6.418, 24.5011, -71.8333) measured on face at (-13.824, 24.5011, -71.8333)
chamfer "Chamfer109" distance 5 distance2 2 3 edges at (-6.418, 25, -83.8104) (-10.121, 25, -83.8104) (-13.824, 25, -83.8104) measured on face at (-13.824, 24.5011, -83.7771) measured on face at (-10.121, 24.5011, -83.7771) measured on face at (-6.418, 24.5011, -83.7771)
chamfer "Chamfer110" distance 5 distance2 2 3 edges at (-13.824, 25, -91.8) (-10.121, 25, -91.8) (-6.418, 25, -91.8) measured on face at (-10.121, 24.5011, -91.8333) measured on face at (-13.824, 24.5011, -91.8333) measured on face at (-6.418, 24.5011, -91.8333)
chamfer "Chamfer111" distance 5 distance2 2 3 edges at (-6.418, 25, -103.8) (-10.121, 25, -103.8) (-13.824, 25, -103.8) measured on face at (-13.824, 24.5011, -103.7667) measured on face at (-10.121, 24.5011, -103.7667) measured on face at (-6.418, 24.5011, -103.7667)
chamfer "Chamfer112" distance 5 distance2 2 3 edges at (-13.824, 25, -123.8) (-10.121, 25, -123.8) (-6.418, 25, -123.8) measured on face at (-6.418, 24.5011, -123.7667) measured on face at (-13.824, 24.5011, -123.7667) measured on face at (-10.121, 24.5011, -123.7667)
chamfer "Chamfer113" distance 5 distance2 2 3 edges at (-13.824, 25, -111.8) (-10.121, 25, -111.8) (-6.418, 25, -111.8) measured on face at (-6.418, 24.5011, -111.8333) measured on face at (-13.824, 24.5011, -111.8333) measured on face at (-10.121, 24.5011, -111.8333)
body "Solid1"
